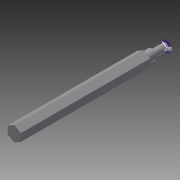
# Autodesk Inventor part: hex rod
Saved by Autodesk Inventor 2015 (Build 190159000, 159)
## iProperties
Created: 2015-01-17
Part Number: hex rod
Material: Generic
Document SubType Name: Modeling
Designer: mastkee16
Density: 1 g/cm^3
Appearance: Default
Author: mastkee16
Autodesk Inventor part; units mm, degrees
ref_plane "YZ Plane" through (0, 0, 0) normal (1, 0, 0) x (0, 1, 0)
ref_plane "XZ Plane" through (0, 0, 0) normal (0, 1, 0) x (-1, 0, 0)
ref_plane "XY Plane" through (0, 0, 0) normal (0, 0, 1) x (1, 0, 0)
sketch "Sketch3" plane through (0, 0, 0) normal (0, 0, 1) x (1, 0, 0)
  circle A0 centre (0, 0) radius 4.7625
  circle A1 centre (0, 0) radius 3.175
  dimension "d4" = 9.525
  dimension "d5" = 6.35
  constraints: 2 centre point, 2 coincident
  measures "d4" diameter of A0
  measures "d5" diameter of A1
extrude "Extrusion2" add sketch "Sketch3" along normal blind 143.51 contours A0 | A1
extrude "Extrusion3" cut sketch "Sketch3" along normal blind 13.2055
sketch "Sketch4" plane through (0, 0, 143.51) normal (0, 0, 1) x (1, 0, 0)
  circle A0 centre (0, 0) radius 3.175 projected
  line L0 (0, -7.1984) -> (-6.234, -3.5992)
  line L1 (-6.234, -3.5992) -> (-6.234, 3.5992)
  line L2 (-6.234, 3.5992) -> (0, 7.1984)
  line L3 (0, 7.1984) -> (6.234, 3.5992)
  line L4 (6.234, 3.5992) -> (6.234, -3.5992)
  line L5 (6.234, -3.5992) -> (0, -7.1984)
  dimension "d10" = 14.3967
  constraints: 12 end point, 1 coincident, 13 other
  measures "d10" distance of L0.start L2.end
extrude "Extrusion4" add sketch "Sketch4" against normal blind 122.6287
body "Solid2"
